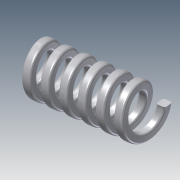
# Autodesk Inventor part: torsion spring
Saved by Autodesk Inventor 2015 (Build 190159000, 159)
## iProperties
Created: 2017-05-07
Part Number: torsion spring
Material: 일반
Document SubType Name: Modeling
Designer: gatew
Density: 1 g/cm^3
Appearance: 기본값
Author: gatew
Autodesk Inventor part; units mm, degrees
ref_plane "YZ Plane" through (0, 0, 0) normal (1, 0, 0) x (0, 1, 0)
ref_plane "XZ Plane" through (0, 0, 0) normal (0, 1, 0) x (-1, 0, 0)
ref_plane "XY Plane" through (0, 0, 0) normal (0, 0, 1) x (1, 0, 0)
sketch "스케치5" plane through (0, 0, 0) normal (1, 0, 0) x (0, 1, 0)
  line L0 (0, 0) -> (-25, 0)
  line L1 (0.5, 5.5) -> (-0.5, 5.5)
  line L2 (-1, 5) -> (-1, 4)
  line L3 (-0.5, 3.5) -> (0.5, 3.5)
  line L4 (1, 4) -> (1, 5)
  line L5 (1, 5.5) -> (-1, 3.5) construction
  line L6 (-1, 5.5) -> (1, 3.5) construction
  arc A0 (-0.5, 5.5) -> (-1, 5) centre (-0.5, 5) ccw
  arc A1 (-1, 4) -> (-0.5, 3.5) centre (-0.5, 4) ccw
  arc A2 (0.5, 3.5) -> (1, 4) centre (0.5, 4) ccw
  arc A3 (1, 5) -> (0.5, 5.5) centre (0.5, 5) ccw
  point P0 (0, 4.5)
  dimension "d29" = 25
  dimension "d30" = 2
  dimension "d31" = 2
  dimension "d32" = 9
  dimension "d41" = 0.5
  dimension "d42" = 0.5
  constraints: 14 end point, 8 point on circle, 8 point on line, 8 tangent, 4 centre point, 2 equal radius, 2 horizontal, 2 midpoint, 2 parallel, 1 perpendicular
  measures "d29" distance of L0.start L0.end
  measures "d30" distance of L6.end L5.end
  measures "d31" distance of L5.end L6.start
  measures "d32" diameter of point (0, 4.5) L0
  measures "d41" radius of A0
  measures "d42" radius of A1
coil "코일3" sketch "스케치5" operation add axis through (0, 0, 0) along (0, -1, 0) pitch 4 turns 6.25 hand right
equation "\"d34\" = d29"
